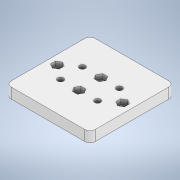
# Autodesk Inventor part: UpperJawSupport
Saved by Autodesk Inventor 2022 (Build 260153000, 153)
## iProperties
Created: 2021-11-03
Part Number: UpperJawSupport
Material: Plástico ABS
Document SubType Name: Modeling
Designer: JK
Density: 1.06 g/cm^3
Appearance: Suave - Blanco
Author: JK
Autodesk Inventor part; units mm, degrees
ref_plane "YZ Plane" through (0, 0, 0) normal (1, 0, 0) x (0, 1, 0)
ref_plane "XZ Plane" through (0, 0, 0) normal (0, 1, 0) x (-1, 0, 0)
ref_plane "XY Plane" through (0, 0, 0) normal (0, 0, 1) x (1, 0, 0)
sketch "Boceto1" plane through (0, 0, 0) normal (0, 1, 0) x (-1, 0, 0)
  line L0 (-38.575, 38.575) -> (38.575, 38.575)
  line L1 (38.575, 38.575) -> (38.575, -38.575)
  line L2 (38.575, -38.575) -> (-38.575, -38.575)
  line L3 (-38.575, -38.575) -> (-38.575, 38.575)
  line L4 (-38.575, 38.575) -> (38.575, -38.575) construction
  line L5 (38.575, 38.575) -> (-38.575, -38.575) construction
  circle A0 centre (30, 0) radius 2.7
  circle A1 centre (-30, 0) radius 2.7
  circle A2 centre (0, 10) radius 2.7
  circle A3 centre (0, -10) radius 2.7
  point P0 (0, 0)
  dimension "d0" = 5.4
  dimension "d1" = 60
  dimension "d3" = 20
  dimension "d4" = 10
  dimension "d5" = 30
  dimension "d6" = 77.15
  dimension "d7" = 77.15
  constraints: 12 end point, 4 centre point, 3 equal radius, 2 midpoint, 2 parallel, 1 horizontal, 1 perpendicular
  measures "d0" diameter of A2
  measures "d1" distance of A1.centre A0.centre
  measures "d3" distance of A3.centre A2.centre
  measures "d4" distance of point (0, 0) A2.centre
  measures "d5" distance of point (0, 0) A0.centre
  measures "d6" distance between parallel lines of L3 L1
  measures "d7" distance of L0.end L1.end
extrude "Extrusión1" add sketch "Boceto1" along normal blind 9.6
sketch "Boceto2" plane through (0, 9.6, 0) normal (0, 1, 0) x (1, 0, 0)
  circle A0 centre (-17, -10) radius 2.7
  circle A1 centre (-17, 10) radius 2.7
  circle A2 centre (17, -10) radius 2.7
  circle A3 centre (17, 10) radius 2.7
  line L0 (38.575, 38.575) -> (-38.575, 38.575) projected
  point P0 (0, 0)
  dimension "d10" = 5.4
  dimension "d11" = 17
  dimension "d13" = 20
  dimension "d14" = 10
  dimension "d15" = 17
  constraints: 4 centre point, 3 equal radius, 2 horizontal alignment, 2 vertical alignment
  measures "d10" diameter of A0
  measures "d11" horizontal distance of A0.centre point (0, 0)
  measures "d13" distance of A0.centre A1.centre
  measures "d14" vertical distance of point (0, 0) A0.centre
  measures "d15" horizontal distance of point (0, 0) A2.centre
extrude "Extrusión2" cut sketch "Boceto2" against normal through all
sketch "Boceto3" plane through (0, 9.6, 0) normal (0, 1, 0) x (1, 0, 0)
  circle A0 centre (-30, 0) radius 2.7 projected
  circle A1 centre (-30, 0) radius 4.05
  line L0 (-30, 4.6765) -> (-25.95, 2.3383)
  line L1 (-25.95, 2.3383) -> (-25.95, -2.3383)
  line L2 (-25.95, -2.3383) -> (-30, -4.6765)
  line L3 (-30, -4.6765) -> (-34.05, -2.3383)
  line L4 (-34.05, -2.3383) -> (-34.05, 2.3383)
  line L5 (-34.05, 2.3383) -> (-30, 4.6765)
  circle A2 centre (0, 10) radius 2.7 projected
  circle A3 centre (0, 10) radius 4.05
  circle A4 centre (0, -10) radius 2.7 projected
  circle A5 centre (0, -10) radius 4.05
  circle A6 centre (30, 0) radius 2.7 projected
  circle A7 centre (30, 0) radius 4.05
  line L6 (4.6765, 10) -> (2.3383, 5.95)
  line L7 (2.3383, 5.95) -> (-2.3383, 5.95)
  line L8 (-2.3383, 5.95) -> (-4.6765, 10)
  line L9 (-4.6765, 10) -> (-2.3383, 14.05)
  line L10 (-2.3383, 14.05) -> (2.3383, 14.05)
  line L11 (2.3383, 14.05) -> (4.6765, 10)
  line L12 (4.6765, -10) -> (2.3383, -14.05)
  line L13 (2.3383, -14.05) -> (-2.3383, -14.05)
  line L14 (-2.3383, -14.05) -> (-4.6765, -10)
  line L15 (-4.6765, -10) -> (-2.3383, -5.95)
  line L16 (-2.3383, -5.95) -> (2.3383, -5.95)
  line L17 (2.3383, -5.95) -> (4.6765, -10)
  line L18 (34.05, -2.3383) -> (30, -4.6765)
  line L19 (30, -4.6765) -> (25.95, -2.3383)
  line L20 (25.95, -2.3383) -> (25.95, 2.3383)
  line L21 (25.95, 2.3383) -> (30, 4.6765)
  line L22 (30, 4.6765) -> (34.05, 2.3383)
  line L23 (34.05, 2.3383) -> (34.05, -2.3383)
  point P0 (0, 0)
  dimension "d18" = 8.1
  constraints: 48 end point, 8 coincident, 4 centre point, 4 tangent, 3 equal radius, 2 horizontal, 1 horizontal alignment, 1 vertical alignment, 52 other
  measures "d18" diameter of A1
extrude "Extrusión3" cut sketch "Boceto3" against normal blind 4.5 contours A0 | A1 | L1 L2 A1 | A1 L0 L1 | A1 L5 L0 | L2 L3 A1 | A1 L4 L5 | L3 L4 A1 | A2 | A3 | A3 L11 L6 | A3 L10 L11 | L6 L7 A3 | A3 L9 L10 | L7 L8 A3 | A3 L8 L9 | A4 | A5 | A5 L17 L12 | A5 L16 L17 | L12 L13 A5 | A5 L15 L16 | L13 L14 A5 | A5 L14 L15 | A6 | A7 | L23 L18 A7 | A7 L22 L23 | A7 L21 L22 | L18 L19 A7 | A7 L20 L21 | L19 L20 A7
fillet "Empalme1" radius 4.635 4 edges at (-38.575, 4.8, 38.575) (38.575, 4.8, 38.575) (38.575, 4.8, -38.575) (-38.575, 4.8, -38.575)
sketch "Boceto4" plane through (0, 0, 0) normal (0, -1, 0) x (1, 0, 0)
  circle A0 centre (-17, 10) radius 2.7 projected
  circle A1 centre (-17, 10) radius 4.05
  line L0 (-19.3383, 14.05) -> (-14.6617, 14.05)
  line L1 (-14.6617, 14.05) -> (-12.3235, 10)
  line L2 (-12.3235, 10) -> (-14.6617, 5.95)
  line L3 (-14.6617, 5.95) -> (-19.3383, 5.95)
  line L4 (-19.3383, 5.95) -> (-21.6765, 10)
  line L5 (-21.6765, 10) -> (-19.3383, 14.05)
  point P0 (0, 0)
  dimension "d22" = 8.1
  constraints: 12 end point, 2 coincident, 1 centre point, 1 horizontal alignment, 1 tangent, 13 other
  measures "d22" diameter of A1
extrude "Extrusión4" cut sketch "Boceto4" against normal blind 4.5 contours A0 | A1 | A1 L1 L2 | A1 L0 L1 | L2 L3 A1 | A1 L5 L0 | L3 L4 A1 | A1 L4 L5
pattern_linear "Patrón rectangular1" count 2 spacing 34 along (1, 0, 0) count 2 spacing 20 along (0, 0, -1) of "Extrusión4"
